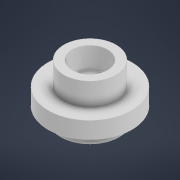
# Autodesk Inventor part: 3
Saved by Autodesk Inventor 2021.2 (Build 252289000, 289)
## iProperties
Created: 2023-09-06
Part Number: 3
Material: Типовые
Document SubType Name: Modeling
Designer: User
Density: 1 g/cm^3
Appearance: По умолчанию
Author: User
Autodesk Inventor part; units mm, degrees
ref_plane "YZ Plane" through (0, 0, 0) normal (1, 0, 0) x (0, 1, 0)
ref_plane "XZ Plane" through (0, 0, 0) normal (0, 1, 0) x (-1, 0, 0)
ref_plane "XY Plane" through (0, 0, 0) normal (0, 0, 1) x (1, 0, 0)
sketch "Эскиз1" plane through (0, 0, 0) normal (0, 0, 1) x (1, 0, 0)
  line L0 (6, 0) -> (12, 0)
  line L1 (12, 0) -> (12, 8)
  line L2 (12, 8) -> (20, 8)
  line L3 (20, 8) -> (20, 0)
  line L4 (20, 0) -> (28, 0)
  line L5 (28, 0) -> (28, 12)
  line L6 (28, 12) -> (40, 12)
  line L7 (40, 12) -> (40, 28)
  line L8 (40, 28) -> (25, 28)
  line L9 (25, 28) -> (25, 50)
  line L10 (25, 50) -> (17, 50)
  line L11 (17, 50) -> (17, 30)
  line L12 (17, 30) -> (6, 30)
  line L13 (6, 30) -> (6, 0)
  line L14 (6, 0) -> (0, 0)
  line L15 (0, 0) -> (0, 22.7372)
  dimension "d0" = 6
  dimension "d1" = 8
  dimension "d2" = 8
  dimension "d4" = 12
  dimension "d5" = 12
  dimension "d7" = 15
  dimension "d8" = 22
  dimension "d10" = 20
  dimension "d11" = 11
  dimension "d12" = 8
  dimension "d13" = 8
  dimension "d14" = 30
  dimension "d15" = 6
  constraints: 32 end point, 11 perpendicular, 2 horizontal, 2 point on line, 1 vertical
  measures "d0" distance of L0.start L0.end
  measures "d1" distance of L0.end L1.end
  measures "d2" distance of L1.end L2.end
  measures "d4" distance of L4.end L5.end
  measures "d5" distance of L5.end L6.end
  measures "d7" distance of L7.end L8.end
  measures "d8" distance of L8.end L9.end
  measures "d10" distance of L10.end L11.end
  measures "d11" distance of L11.end L12.end
  measures "d12" distance of L9.end L10.end
  measures "d13" distance of L3.end L4.end
  measures "d14" distance of L12.end L0.start
  measures "d15" distance of L0.start L14.end
revolve "Вращение1" add sketch "Эскиз1" angle 360 about axis through (0, 0, 0) along (0, 1, 0)
